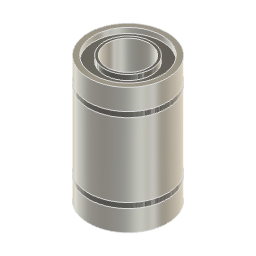
_Linear Ball bearings.70847623-6915-440d-9f91-3413167815d5 (Autodesk Fusion 360 design; units mm, degrees)
Autodesk Fusion 360 part; units mm, degrees
note: some values were not read from the file. Chosen so that the rebuilt part matches the saved one: that a step has no effect.
sketch "Sketch1" plane through (0, 0, 0) normal (0, 0, 1) x (1, 0, 0)
  circle A0 centre (0, 0) radius 4
  circle A1 centre (0, 0) radius 7.5
  dimension "d1" = 8
  dimension "d2" = 15
  constraint coincident A0.centre A1.centre
  measures "d1" diameter of A0
  measures "d2" diameter of A1
extrude "Extrude1" add sketch "Sketch1" along normal blind 24
sketch "Sketch2" plane through (0, 0, 24) normal (0, 0, 1) x (-1, 0, 0)
  circle A0 centre (0, 0) radius 4
  circle A1 centre (0, 0) radius 7.5
  circle A2 centre (0, 0) radius 6.5
  circle A3 centre (0, 0) radius 4.5
  dimension "d5" = -1
  dimension "d6" = 0.5
extrude "Extrude2" cut sketch "Sketch2" against normal blind 1 contours A2
ref_plane "WorkPlane1" through (0, 0, 12) normal (0, 0, 1) x (1, 0, 0)
mirror "Mirror1" about plane through (0, 0, 12) normal (0, 0, 1) of "Extrude2"
ref_plane "WorkPlane2" through (0, 0, 4) normal (0, 0, -1) x (-1, 0, 0)
ref_plane "WorkPlane3" through (0, 0, 5) normal (0, 0, -1) x (-1, 0, 0)
split_face "SplitFace1" [no effect]
mirror "Mirror2" [no effect]
